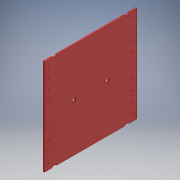
# Autodesk Inventor part: Backplane_PCB
Saved by Autodesk Inventor 2018 (Build 220112000, 112)
## iProperties
Created: 2018-07-04
Part Number: Backplane_PCB
Material: Epoxy Resin
Document SubType Name: Modeling
Designer: Bradley
Density: 1.14 g/cm^3
Appearance: Smooth - Red
Mass: 8.06113 g
Surface Area: 145.658 cm^2
Volume: 7.07117 cm^3
Author: Bradley
Autodesk Inventor part; units mm, degrees
ref_plane "YZ Plane" through (0, 0, 0) normal (1, 0, 0) x (0, 1, 0)
ref_plane "XZ Plane" through (0, 0, 0) normal (0, 1, 0) x (-1, 0, 0)
ref_plane "XY Plane" through (0, 0, 0) normal (0, 0, 1) x (1, 0, 0)
sketch "Sketch1" plane through (0, 0, 0) normal (1, 0, 0) x (0, 1, 0)
  line L0 (-41.4, -43) -> (41.4, -43)
  line L1 (41.4, -43) -> (41.4, 43)
  line L2 (41.4, 43) -> (-41.4, 43)
  line L3 (-41.4, 43) -> (-41.4, -43)
  line L4 (-41.4, -43) -> (41.4, 43) construction
  line L5 (41.4, -43) -> (-41.4, 43) construction
  point P0 (0, 0)
  dimension "d0" = 82.8
  dimension "d1" = 86
  constraints: 12 end point, 2 midpoint, 2 parallel, 1 horizontal, 1 perpendicular
  measures "d0" distance of L2.end L1.end
  measures "d1" distance of L1.end L0.end
extrude "Extrusion1" add sketch "Sketch1" along normal mid plane 1
sketch "Sketch2" plane through (0.5, 0, 0) normal (1, 0, 0) x (0, 0, -1)
  line L0 (0, -15) -> (0, 15) construction
  point P0 (0, 0)
  point P1 (0, 0)
  dimension "d4" = 30
  constraints: 3 coincident, 2 end point, 1 midpoint, 1 vertical
  measures "d4" distance of L0.start L0.end
hole "Hole1" at (0.5, -15, 0) at (0.5, 15, 0) direction (-1, 0, 0) diameter 3.3 end through all clearance for "Flat Head Machine Screw" size "M3" standard "Ansi Metric M Profile"
sketch "Sketch3" plane through (0.5, 0, 0) normal (1, 0, 0) x (0, 0, -1)
  circle A0 centre (37.5, -38.3) radius 0.725
  circle A1 centre (37.5, 38.3) radius 0.525
  line L0 (37.5, -38.3) -> (37.5, 38.3) construction
  circle A2 centre (-10.5, -38.3) radius 0.725
  circle A3 centre (-10.5, 38.3) radius 0.525
  circle A4 centre (0, -15) radius 1.65 projected
  circle A5 centre (0, 15) radius 1.65 projected
  line L1 (43, -41.4) -> (43, 41.4) projected
  line L2 (43, 41.4) -> (-43, 41.4) projected
  line L3 (-43, 41.4) -> (-43, -41.4) projected
  line L4 (-43, -41.4) -> (43, -41.4) projected
  circle A6 centre (-19.5, -38.3) radius 0.725
  circle A7 centre (-19.5, 38.3) radius 0.525
  circle A8 centre (28.5, 38.3) radius 0.525
  circle A9 centre (28.5, -38.3) radius 0.725
  circle A10 centre (-28.5, -38.3) radius 0.725
  circle A11 centre (-28.5, 38.3) radius 0.525
  circle A12 centre (19.5, 38.3) radius 0.525
  circle A13 centre (19.5, -38.3) radius 0.725
  circle A14 centre (-37.5, -38.3) radius 0.725
  circle A15 centre (-37.5, 38.3) radius 0.525
  circle A16 centre (10.5, 38.3) radius 0.525
  circle A17 centre (10.5, -38.3) radius 0.725
  point P0 (0, 0)
  point P1 (37.5, 0)
  dimension "d12" = 1.05
  dimension "d13" = 1.45
  dimension "d14" = 76.6
  dimension "d17" = 9
  dimension "d22" = 21
  dimension "d23" = 10.5
  constraints: 16 centre point, 3 horizontal alignment, 2 end point, 2 equal radius, 1 horizontal, 1 midpoint, 1 vertical, 1 vertical alignment, 24 other
  measures "d12" diameter of A1
  measures "d13" diameter of A0
  measures "d14" distance of L0.start L0.end
  measures "d17" distance of A2.centre A6.centre
  measures "d22" distance of A17.centre A2.centre
  measures "d23" horizontal distance of point (0, 0) A17.centre
extrude "Extrusion2" cut sketch "Sketch3" against normal through all contours A0 | A1 | A2 | A3 | A6 | A7 | A8 | A9 | A10 | A11 | A12 | A13 | A14 | A15 | A16 | A17
sketch "Sketch4" plane through (0.5, 0, 0) normal (1, 0, 0) x (0, 0, -1)
  circle A0 centre (-37.5, -38.3) radius 0.725 projected
  circle A1 centre (-28.5, -38.3) radius 0.725 projected
  circle A2 centre (-19.5, -38.3) radius 0.725 projected
  circle A3 centre (37.5, -38.3) radius 0.725 projected
  circle A4 centre (-37.5, 38.3) radius 0.525 projected
  circle A5 centre (-28.5, 38.3) radius 0.525 projected
  circle A6 centre (-19.5, 38.3) radius 0.525 projected
  circle A7 centre (37.5, 38.3) radius 0.525 projected
  circle A8 centre (-10.5, 38.3) radius 0.525 projected
  circle A9 centre (28.5, 38.3) radius 0.525 projected
  circle A10 centre (19.5, 38.3) radius 0.525 projected
  circle A11 centre (10.5, 38.3) radius 0.525 projected
  circle A12 centre (-10.5, -38.3) radius 0.725 projected
  circle A13 centre (28.5, -38.3) radius 0.725 projected
  circle A14 centre (19.5, -38.3) radius 0.725 projected
  circle A15 centre (10.5, -38.3) radius 0.725 projected
  circle A16 centre (0, -15) radius 1.65 projected
  circle A17 centre (0, 15) radius 1.65 projected
  line L0 (43, -41.4) -> (43, 41.4) projected
  line L1 (43, 41.4) -> (-43, 41.4) projected
  line L2 (-43, 41.4) -> (-43, -41.4) projected
  line L3 (-43, -41.4) -> (43, -41.4) projected
  line L4 (-43, 41.4) -> (-43, -41.4) projected
  arc A18 (-43, -34.7361) -> (-43, -30.2639) centre (-45, -32.5) ccw
  arc A19 (-43, 30.2639) -> (-43, 34.7361) centre (-45, 32.5) ccw
  line L5 (43, -41.4) -> (43, 41.4) projected
  arc A20 (43, -30.2639) -> (43, -34.7361) centre (45, -32.5) ccw
  arc A21 (43, 34.7361) -> (43, 30.2639) centre (45, 32.5) ccw
  line L6 (-45, -32.5) -> (45, -32.5) construction
  line L7 (-45, -32.5) -> (-45, 32.5) construction
  point P0 (0, 0)
  point P1 (0, -32.5)
  point P2 (-45, 0)
  dimension "d26" = 65
  dimension "d27" = 3
  dimension "d28" = 90
  constraints: 8 point on circle, 8 point on line, 4 centre point, 4 end point, 3 equal radius, 2 horizontal alignment, 2 midpoint, 2 vertical alignment, 1 horizontal, 1 vertical
  measures "d26" distance of L6.start L7.end
  measures "d27" radius of A18
  measures "d28" distance of L6.start L6.end
extrude "Extrusion3" cut sketch "Sketch4" against normal through all contours A20 L0 | L2 A18 | A21 L0 | L2 A19
equation "\"d23\" = 0.5 * d22"
body "Solid1"
